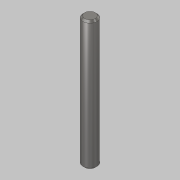
# Autodesk Inventor part: ShaftLegUpper
Saved by Autodesk Inventor 2019.2 (Build 232265000, 265)
## iProperties
Created: 2019-02-05
Part Number: ShaftLegUpper
Material: Stahl, Legierung
Document SubType Name: Modeling
Designer: Lion
Density: 7.73 g/cm^3
Appearance: Halbpoliert
Author: Lion
Autodesk Inventor part; units mm, degrees
ref_plane "YZ Plane" through (0, 0, 0) normal (1, 0, 0) x (0, 1, 0)
ref_plane "XZ Plane" through (0, 0, 0) normal (0, 1, 0) x (-1, 0, 0)
ref_plane "XY Plane" through (0, 0, 0) normal (0, 0, 1) x (1, 0, 0)
derived "Shaft1.ipt"
sketch "Skizze1" plane through (0, 0, 0) normal (0, 1, 0) x (-1, 0, 0)
  circle A0 centre (0, 0) radius 1
extrude "Extrusion1" add sketch "Skizze1" along normal blind 18.5
chamfer "Fase1" distance 0.25 angle 45 2 edges at (1, 18.5, 0) (1, 0, 0)
